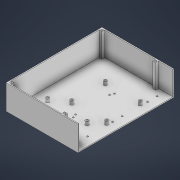
# Autodesk Inventor part: Grundplatte_vorne
Saved by Autodesk Inventor 2021 (Build 250183000, 183)
## iProperties
Created: 2021-01-26
Part Number: Grundplatte_vorne
Material: Generisch
Document SubType Name: Modeling
Designer: Ctroi
Density: 1 g/cm^3
Appearance: Vorgabe
Author: Ctroi
## iProperties of the stored document _3D-Druck.ipt
Created: 2021-02-01
Part Number: _3D-Druck
Material: Generisch
Document SubType Name: Modeling
Designer: Ctroi
Density: 1 g/cm^3
Appearance: Vorgabe
Author: Ctroi
Autodesk Inventor part; units mm, degrees
ref_plane "YZ Plane" through (0, 0, 0) normal (1, 0, 0) x (0, 1, 0)
ref_plane "XZ Plane" through (0, 0, 0) normal (0, 1, 0) x (-1, 0, 0)
ref_plane "XY Plane" through (0, 0, 0) normal (0, 0, 1) x (1, 0, 0)
sketch "Skizze1" plane through (0, 0, 0) normal (0, 1, 0) x (-1, 0, 0)
  line L0 (0, -140) -> (0, 140) projected
  line L1 (-105, 0) -> (105, 0) projected
  line L2 (75, -100) -> (-75, -100)
  line L3 (-75, -100) -> (-75, 100)
  line L4 (-75, 100) -> (75, 100)
  line L5 (75, 100) -> (75, -100)
  point P0 (0, 0)
  dimension "d0" = 150
  dimension "d1" = 200
  constraints: 8 end point, 2 parallel, 1 horizontal, 1 perpendicular, 2 other
  measures "d0" distance of L3.end L4.end
  measures "d1" distance of L2.end L3.end
extrude "Extrusion1" add sketch "Skizze1" along normal blind 2
sketch "Skizze2" plane through (0, 2, 0) normal (0, 1, 0) x (1, 0, 0)
  circle A0 centre (57.5, 82.5) radius 1.6
  line L0 (75, -100) -> (75, 100) projected
  line L1 (75, 100) -> (-75, 100) projected
  circle A1 centre (57.5, 62.5) radius 1.6
  line L2 (105, 0) -> (-105, 0) projected
  circle A2 centre (57.5, -82.5) radius 1.6
  circle A3 centre (57.5, -62.5) radius 1.6
  point P0 (0, 0)
  dimension "d4" = 3.2
  dimension "d5" = 17.5
  dimension "d6" = 17.5
  dimension "d7" = 3.2
  dimension "d8" = 20
  dimension "d9" = 17.5
  constraints: 4 centre point, 2 symmetric about line, 2 other
  measures "d4" diameter of A0
  measures "d5" distance from line of L0 A0.centre
  measures "d6" distance from line of L1 A0.centre
  measures "d7" diameter of A1
  measures "d8" distance of A0.centre A1.centre
  measures "d9" distance from line of L0 A1.centre
extrude "Extrusion2" cut sketch "Skizze2" against normal up to surface (2 mm away)
sketch "Skizze4" plane through (0, 2, 0) normal (0, 1, 0) x (1, 0, 0)
  line L0 (-75, -100) -> (75, -100) projected
  line L1 (-75, 100) -> (-75, -100) projected
  line L2 (75, -100) -> (-75, -100)
  line L3 (-75, -100) -> (-75, -98)
  line L4 (-75, -98) -> (75, -98)
  line L5 (75, -98) -> (75, -100)
  line L6 (75, 100) -> (-75, 100) projected
  line L7 (75, 100) -> (-75, 100)
  line L8 (-75, 100) -> (-75, 98)
  line L9 (-75, 98) -> (75, 98)
  line L10 (75, 98) -> (75, 100)
  line L11 (75, -98) -> (39, -98)
  line L12 (39, -98) -> (39, -92)
  line L13 (39, -92) -> (45, -92)
  line L14 (75, 98) -> (39, 98)
  line L15 (39, 98) -> (39, 92)
  line L16 (39, 92) -> (45, 92)
  line L17 (-75, -98) -> (-73, -98)
  line L18 (-73, -98) -> (-73, 98)
  line L19 (-73, 98) -> (-75, 98)
  line L20 (-75, 98) -> (-75, -98)
  line L21 (-73, 98) -> (-67, 98)
  line L22 (-67, 98) -> (-67, 92)
  line L23 (-67, 92) -> (-73, 92)
  line L24 (-73, 92) -> (-73, 98)
  line L25 (-73, -98) -> (-67, -98)
  line L26 (-67, -98) -> (-67, -92)
  line L27 (-67, -92) -> (-73, -92)
  line L28 (-73, -92) -> (-73, -98)
  line L29 (45, -92) -> (45, -98)
  line L30 (75, -100) -> (75, 100) projected
  line L31 (45, 98) -> (45, 92)
  point P0 (0, 0)
  point P1 (75, 92)
  point P2 (39, -98)
  point P3 (39, -98)
  dimension "d18" = 2
  dimension "d19" = 2
  dimension "d21" = 6
  dimension "d23" = 6
  dimension "d24" = 2
  dimension "d25" = 6
  dimension "d26" = 6
  dimension "d27" = 6
  dimension "d28" = 6
  dimension "d130" = 6
  dimension "d131" = 30
  dimension "d132" = 6
  dimension "d133" = 30
  constraints: 56 end point, 12 parallel, 9 perpendicular, 7 horizontal, 5 point on line
  measures "d18" distance of L2.end L3.end
  measures "d19" distance of L8.end L7.end
  measures "d21" distance of L11.end L12.end
  measures "d23" distance of L15.end L14.end
  measures "d24" distance of L19.end L18.end
  measures "d25" distance of L22.end L23.end
  measures "d26" distance of L21.end L22.end
  measures "d27" distance of L27.end L26.end
  measures "d28" distance of L26.end L25.end
  measures "d130" distance between parallel lines of L12 L29
  measures "d131" distance between parallel lines of L30 L29
  measures "d132" distance between parallel lines of L31 L15
  measures "d133" distance between parallel lines of L30 L31
extrude "Extrusion4" add sketch "Skizze4" along normal blind 50 contours L1 L4 L5 L0 | L1 L9 L18 L4 | L1 L6 L10 L9 | L18 L27 L26 L4 | L4 L12 L13 L29 | L9 L22 L23 L18 | L31 L16 L15 L9
sketch "Skizze5" plane through (0, 2, 0) normal (0, 1, 0) x (1, 0, 0)
  circle A0 centre (55, 50) radius 3.5
  circle A1 centre (55, -20) radius 3.5
  line L0 (-105, 0) -> (105, 0) projected
  line L1 (105, 0) -> (-105, 0) projected
  line L2 (75, -98) -> (75, 98) projected
  circle A2 centre (-18, -20) radius 3.5
  circle A3 centre (-18, 50) radius 3.5
  line L3 (75, 100) -> (-75, 100) projected
  circle A4 centre (35.2743, -41.2) radius 3.5
  circle A5 centre (-47.2757, -41.2) radius 3.5
  circle A6 centre (-40.9257, -89.46) radius 3.5
  circle A7 centre (34.0043, -89.46) radius 3.5
  line L4 (-75, -100) -> (75, -100) projected
  line L5 (-75, 100) -> (-75, -100) projected
  point P0 (0, 0)
  point P1 (75, 92)
  dimension "d31" = 7
  dimension "d32" = 7
  dimension "d35" = 20
  dimension "d36" = 20
  dimension "d37" = 7
  dimension "d38" = 73
  dimension "d40" = 7
  dimension "d42" = 73
  dimension "d68" = 70
  dimension "d69" = 70
  dimension "d70" = 50
  dimension "d73" = 50
  dimension "d74" = 7
  dimension "d75" = 7
  dimension "d83" = 7
  dimension "d86" = 7
  dimension "d110" = 10.54
  dimension "d111" = 40.9957
  dimension "d113" = 58.8
  dimension "d114" = 39.7257
  dimension "d115" = 10.54
  dimension "d116" = 34.0743
  dimension "d117" = 27.7243
  dimension "d118" = 58.8
  constraints: 8 centre point
  measures "d31" diameter of A0
  measures "d32" diameter of A1
  measures "d35" distance from line of L2 A0.centre
  measures "d36" distance from line of L2 A1.centre
  measures "d37" diameter of A2
  measures "d38" distance of A1.centre A2.centre
  measures "d40" diameter of A3
  measures "d42" distance of A0.centre A3.centre
  measures "d68" distance of A0.centre A1.centre
  measures "d69" distance of A3.centre A2.centre
  measures "d70" distance from line of L0 A0.centre
  measures "d73" distance from line of L3 A3.centre
  measures "d74" diameter of A4
  measures "d75" diameter of A5
  measures "d83" diameter of A6
  measures "d86" diameter of A7
  measures "d110" distance from line of L4 A7.centre
  measures "d111" distance from line of L2 A7.centre
  measures "d113" distance from line of L4 A4.centre
  measures "d114" distance from line of L2 A4.centre
  measures "d115" distance from line of L4 A6.centre
  measures "d116" distance from line of L5 A6.centre
  measures "d117" distance from line of L5 A5.centre
  measures "d118" distance from line of L4 A5.centre
extrude "Extrusion5" add sketch "Skizze5" along normal blind 7
sketch "Skizze6" plane through (-18, 9, -50) normal (0, 1, 0) x (1, 0, 0)
  circle A0 centre (0, 0) radius 2
  circle A1 centre (73, 0) radius 3.5 projected
  circle A2 centre (73, 0) radius 2
  circle A3 centre (0, -70) radius 2
  circle A4 centre (0, -70) radius 3.5 projected
  circle A5 centre (73, -70) radius 3.5 projected
  circle A6 centre (73, -70) radius 2
  circle A7 centre (52.0043, -139.46) radius 2
  circle A8 centre (52.0043, -139.46) radius 3.5 projected
  circle A9 centre (53.2743, -91.2) radius 2
  circle A10 centre (53.2743, -91.2) radius 3.5 projected
  circle A11 centre (-29.2757, -91.2) radius 2
  circle A12 centre (-29.2757, -91.2) radius 3.5 projected
  circle A13 centre (-22.9257, -139.46) radius 2
  circle A14 centre (-22.9257, -139.46) radius 3.5 projected
  dimension "d45" = 4
  dimension "d46" = 4
  dimension "d47" = 4
  dimension "d48" = 0
  dimension "d49" = 4
  dimension "d50" = 73
  dimension "d51" = 70
  dimension "d96" = 4
  dimension "d97" = 0
  dimension "d98" = 0
  dimension "d99" = 4
  dimension "d100" = 0
  dimension "d101" = 0
  dimension "d102" = 4
  dimension "d103" = 0
  dimension "d104" = 4
  dimension "d105" = 0
  constraints: 8 centre point, 2 coincident
  measures "d45" diameter of A0
  measures "d46" diameter of A2
  measures "d47" diameter of A3
  measures "d48" distance of A4.centre A3.centre
  measures "d49" diameter of A6
  measures "d50" distance of A2.centre A0.centre
  measures "d51" distance of A3.centre A0.centre
  measures "d96" diameter of A7
  measures "d97" distance of A8.centre A7.centre
  measures "d98" distance of A8.centre A7.centre
  measures "d99" diameter of A9
  measures "d100" distance of A10.centre A9.centre
  measures "d101" distance of A10.centre A9.centre
  measures "d102" diameter of A11
  measures "d103" distance of A12.centre A11.centre
  measures "d104" diameter of A13
  measures "d105" distance of A14.centre A13.centre
extrude "Extrusion6" cut sketch "Skizze6" against normal blind 5 contours A0 | A2 | A3 | A6 | A7 | A9 | A11 | A13
sketch "Skizze7" plane through (0, 52, 0) normal (0, 1, 0) x (1, 0, 0)
  circle A0 centre (42, -95) radius 2
  circle A1 centre (-70, -95) radius 2
  circle A2 centre (-70, 95) radius 2
  circle A3 centre (42, 95) radius 2
  line L0 (39, 98) -> (39, 92) projected
  line L1 (39, 92) -> (45, 92) projected
  line L2 (39, -92) -> (39, -98) projected
  line L3 (45, -92) -> (39, -92) projected
  line L4 (-67, -98) -> (-67, -92) projected
  line L5 (-67, -92) -> (-73, -92) projected
  line L6 (-67, 92) -> (-67, 98) projected
  line L7 (-73, 92) -> (-67, 92) projected
  line L8 (45, -98) -> (45, -92) projected
  line L9 (45, 92) -> (45, 98) projected
  point P0 (0, 0)
  point P1 (75, 92)
  point P2 (75, -92)
  dimension "d54" = 4
  dimension "d55" = 4
  dimension "d56" = 4
  dimension "d57" = 4
  dimension "d59" = 3
  dimension "d61" = 3
  dimension "d62" = 3
  dimension "d63" = 3
  dimension "d64" = 3
  dimension "d65" = 3
  dimension "d134" = 3
  dimension "d135" = 3
  constraints: 4 centre point
  measures "d54" diameter of A0
  measures "d55" diameter of A1
  measures "d56" diameter of A2
  measures "d57" diameter of A3
  measures "d59" distance from line of L1 A3.centre
  measures "d61" distance from line of L3 A0.centre
  measures "d62" distance from line of L4 A1.centre
  measures "d63" distance from line of L5 A1.centre
  measures "d64" distance from line of L6 A2.centre
  measures "d65" distance from line of L7 A2.centre
  measures "d134" distance from line of L8 A0.centre
  measures "d135" distance from line of L9 A3.centre
extrude "Extrusion7" cut sketch "Skizze7" against normal blind 5
sketch "Skizze8" plane through (0, 2, 0) normal (0, 1, 0) x (1, 0, 0)
  circle A0 centre (57, 10) radius 1.6
  line L0 (105, 0) -> (-105, 0) projected
  line L1 (75, -98) -> (75, 98) projected
  circle A1 centre (57, -10) radius 1.6
  circle A2 centre (8.109, 42.961) radius 1.6
  circle A3 centre (5.373, 35.444) radius 1.6
  circle A4 centre (8.109, -42.961) radius 1.6
  circle A5 centre (5.373, -35.444) radius 1.6
  point P0 (0, 0)
  point P1 (75, -92)
  point P2 (75, 92)
  dimension "d119" = 3.2
  dimension "d120" = 18
  dimension "d121" = 10
  dimension "d122" = 3.2
  dimension "d123" = 3.2
  dimension "d124" = 66.891
  dimension "d125" = 69.627
  dimension "d126" = 42.961
  dimension "d127" = 35.444
  constraints: 6 centre point, 3 symmetric about line, 3 other
  measures "d119" diameter of A0
  measures "d120" distance from line of L1 A0.centre
  measures "d121" distance from line of L0 A0.centre
  measures "d122" diameter of A2
  measures "d123" diameter of A3
  measures "d124" distance from line of A2.centre L1
  measures "d125" distance from line of L1 A3.centre
  measures "d126" distance from line of L0 A2.centre
  measures "d127" distance from line of L0 A3.centre
extrude "Extrusion8" cut sketch "Skizze8" against normal up to surface (2 mm away)
equation "\"d43\" = d83"
